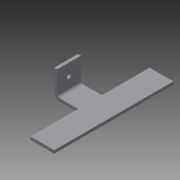
# Autodesk Inventor part: Cylinder Mount 2
Saved by Autodesk Inventor 2013 (Build 170138000, 138)
## iProperties
Created: 2013-01-26
Part Number: Cylinder Mount 2
Material: Generic
Document SubType Name: Sheet Metal
Designer: actoennies
Density: 1 g/cm^3
Sheet Metal Rule: Default
Mass: 16.1985 g
Surface Area: 118.429 cm^2
Volume: 16.1985 cm^3
Author: actoennies
Autodesk Inventor part; units mm, degrees
ref_plane "YZ Plane" through (0, 0, 0) normal (1, 0, 0) x (0, 1, 0)
ref_plane "XZ Plane" through (0, 0, 0) normal (0, 1, 0) x (-1, 0, 0)
ref_plane "XY Plane" through (0, 0, 0) normal (0, 0, 1) x (1, 0, 0)
sketch "Sketch1" plane through (0, 0, 0) normal (1, 0, 0) x (0, 1, 0)
  line L0 (0, 0) -> (25.4, 0)
  line L1 (25.4, 0) -> (25.4, 25.4)
  line L2 (25.4, 25.4) -> (0, 25.4)
  line L3 (0, 25.4) -> (0, 0)
  dimension "d0" = 25.4
  dimension "d2" = 25.4
  measures "d0" distance of L1.end L2.end
  measures "d2" distance of L0.end L1.end
extrude "Plate1" add sketch "Sketch1" along normal blind 3.175
sketch "Sketch2" plane through (3.175, 0, 0) normal (0, -1, 0) x (1, 0, 0)
  line L0 (0, 25.4) -> (0, 0)
  line L1 (0, 0) -> (22.225, 0)
  line L2 (22.225, 0) -> (22.225, 25.4)
  line L3 (22.225, 25.4) -> (0, 25.4)
  constraints: 6 end point, 1 horizontal, 1 perpendicular, 1 vertical
edge flange "Flange1" height 25.4 angle 90 thickness 3.175 bend radius 3.175 thickness toward (0, -1, 0) relief straight relief width 3.175 relief depth 1.5875 edges at (3.175, 0, 12.7) wall of the first edge with corners at (3.175, 0, 25.4) (3.175, 0, 0) (25.4, 0, 0) (25.4, 0, 25.4)
bend "Bend1"
corner "Corner1"
sketch "Sketch3" plane through (25.4, 0, 25.4) normal (0, 1, 0) x (1, 0, 0)
  line L0 (0, 0) -> (0, 25.4)
  line L1 (0, 25.4) -> (-19.05, 25.4)
  line L2 (0, 0) -> (0, -19.05)
  line L3 (0, -19.05) -> (25.4, -19.05)
  line L4 (25.4, -19.05) -> (25.4, 136.525)
  line L5 (25.4, 136.525) -> (0, 136.525)
  line L6 (0, 136.525) -> (0, 25.4)
  point P0 (-25.4, 25.4)
  dimension "d14" = 19.05
  dimension "d15" = 25.4
  dimension "d16" = 155.575
  measures "d14" distance of L0.start L2.end
  measures "d15" distance of L2.end L3.end
  measures "d16" distance of L3.end L4.end
sheet face with bend "Face2" sketch "Sketch3" thickness 3.175 toward (0, -1, 0) bend radius 3.175 relief straight relief width 3.175 relief depth 1.5875
bend "Bend2"
sketch "Sketch4" plane through (0, 0, 0) normal (-1, 0, 0) x (0, 0, 1)
  line L0 (25.4, 25.4) -> (25.4, 3.175) projected
  line L1 (0, 25.4) -> (25.4, 25.4) projected
  circle A0 centre (12.7, 12.7) radius 2.286
  point P0 (0, 0)
  dimension "d22" = 4.572
  dimension "d23" = 12.7
  dimension "d24" = 12.7
  constraints: 1 centre point
  measures "d22" diameter of A0
  measures "d23" distance from line of L1 A0.centre
  measures "d24" distance from line of L0 A0.centre
extrude "Cut1" cut sketch "Sketch4" against normal blind 3.175
sketch "Sketch5" plane through (6.35, 0, 25.4) normal (0, 1, 0) x (1, 0, 0)
  line L0 (19.05, -19.05) -> (44.45, -19.05) projected
  line L1 (44.45, -19.05) -> (44.45, 136.525) projected
  line L2 (44.45, 136.525) -> (19.05, 136.525) projected
  circle A0 centre (31.75, -6.35) radius 3.3782
  circle A1 centre (31.75, 123.825) radius 3.3782
  point P0 (-6.35, 25.4)
  dimension "d27" = 6.7564
  dimension "d28" = 12.7
  dimension "d29" = 12.7
  dimension "d30" = 6.7564
  dimension "d31" = 12.7
  dimension "d32" = 12.7
  constraints: 2 centre point
  measures "d27" diameter of A0
  measures "d28" distance from line of L1 A0.centre
  measures "d29" distance from line of L0 A0.centre
  measures "d30" diameter of A1
  measures "d31" distance from line of L2 A1.centre
  measures "d32" distance from line of L1 A1.centre
extrude "Cut2" cut sketch "Sketch5" against normal blind 3.175
equation "\"d25\" = Thickness"
equation "\"d33\" = Thickness"
equation "\"d4\" = BendReliefWidth"
equation "\"d5\" = BendReliefDepth"
equation "\"d6\" = MinimumRemnant"
equation "\"d7\" = BendRadius"
equation "\"d10\" = BendRadius"
equation "\"d11\" = CornerReliefSize"
equation "\"d12\" = GapSize"
equation "\"d13\" = JacobiRadiusSize"
equation "\"d17\" = BendRadius"
equation "\"d18\" = BendReliefWidth"
equation "\"d20\" = MinimumRemnant"
equation "\"d19\" = BendReliefDepth"
equation "\"d21\" = BendRadius"
equation "\"BendRadius\" = Thickness"
equation "\"BendReliefWidth\" = Thickness"
equation "\"BendReliefDepth\" = 0.5 * Thickness"
equation "\"CornerReliefSize\" = 4 * Thickness"
equation "\"MinimumRemnant\" = 2 * Thickness"
equation "\"TransitionRadius\" = BendRadius"
equation "\"JacobiRadiusSize\" = BendRadius"
equation "\"GapSize\" = Thickness"
equation "\"d3\" = BendRadius"
equation "\"Thickness\" = 3.175"
body "Solid1"
